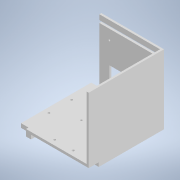
# Autodesk Inventor part: Quarter 3
Saved by Autodesk Inventor 2020.2 (Build 242310000, 310)
## iProperties
Created: 2020-01-17
Part Number: Quarter 3
Material: Generic
Document SubType Name: Modeling
Designer: ColinP
Density: 1 g/cm^3
Appearance: Default
Author: ColinP
Autodesk Inventor part; units mm, degrees
ref_plane "YZ Plane" through (0, 0, 0) normal (1, 0, 0) x (0, 1, 0)
ref_plane "XZ Plane" through (0, 0, 0) normal (0, 1, 0) x (-1, 0, 0)
ref_plane "XY Plane" through (0, 0, 0) normal (0, 0, 1) x (1, 0, 0)
sketch "Sketch1" plane through (0, 0, 0) normal (0, 1, 0) x (-1, 0, 0)
  line L0 (0, 0) -> (125, 0)
  line L1 (125, 0) -> (125, 150)
  line L2 (125, 150) -> (0, 150)
  line L3 (0, 150) -> (0, 0)
  dimension "d0" = 125
  dimension "d1" = 150
  constraints: 8 end point, 2 parallel, 1 horizontal, 1 perpendicular
  measures "d0" distance of L2.end L1.end
  measures "d1" distance of L1.end L0.end
extrude "Extrusion1" add sketch "Sketch1" along normal blind 10
sketch "Sketch2" plane through (0, 10, 0) normal (0, 1, 0) x (1, 0, 0)
  line L0 (-125, -150) -> (0, -150) projected
  line L1 (0, -150) -> (-4, -150)
  line L2 (-4, -150) -> (-4, -4)
  line L3 (-4, -4) -> (-125, -4)
  line L4 (-125, 0) -> (-125, -150) projected
  line L5 (0, -150) -> (0, 0) projected
  line L6 (0, 0) -> (-125, 0) projected
  line L7 (-125, 0) -> (-125, -150) projected
  line L8 (-125, -150) -> (0, -150) projected
  dimension "d4" = 4
  dimension "d5" = 146
  constraints: 6 end point, 2 perpendicular, 2 point on line
  measures "d4" distance of L0.end L1.end
  measures "d5" distance of L1.end L2.end
extrude "Extrusion2" add sketch "Sketch2" along normal blind 125 contours L2 L3 L4 L6 L5 L0
sketch "Sketch4" plane through (-125, 10, 4) normal (0, 0, 1) x (1, 0, 0)
  line L0 (0, -10) -> (0, 0) projected
  line L1 (0, 0) -> (0, 20)
  line L2 (0, -10) -> (0, 125) projected
  line L3 (0, 20) -> (20, 20)
  line L4 (20, 20) -> (86, 20)
  line L5 (86, 20) -> (86, 47)
  line L6 (86, 47) -> (20, 47)
  line L7 (20, 47) -> (20, 20)
  line L8 (20, 47) -> (20, 67)
  line L9 (20, 67) -> (20, 90)
  line L10 (20, 90) -> (20, 67)
  line L11 (20, 67) -> (81.6, 67)
  point P0 (125, -10)
  point P1 (0, -5)
  dimension "d11" = 20
  dimension "d12" = 20
  dimension "d13" = 66
  dimension "d14" = 27
  dimension "d15" = 20
  dimension "d55" = 23
  dimension "d56" = 61.6
  constraints: 20 end point, 3 horizontal, 3 perpendicular, 2 point on line, 1 collinear, 1 vertical
  measures "d11" distance of L0.end L1.end
  measures "d12" distance of L1.end L3.end
  measures "d13" distance of L3.end L4.end
  measures "d14" distance of L4.end L5.end
  measures "d15" distance of L6.end L8.end
  measures "d55" distance of L8.end L9.end
  measures "d56" distance of L8.end L11.end
extrude "Extrusion4" cut sketch "Sketch4" against normal blind 10
sketch "Sketch7" plane through (-125, 0, 150) normal (0, 0, 1) x (1, 0, 0)
  line L0 (125, 0) -> (0, 0) projected
  line L1 (125, 0) -> (125, 5)
  line L2 (125, 0) -> (125, 135) projected
  line L3 (125, 5) -> (10, 5)
  line L4 (10, 5) -> (10, 0)
  line L5 (10, 0) -> (125, 0)
  dimension "d32" = 5
  dimension "d33" = 115
  constraints: 8 end point, 2 perpendicular, 1 parallel, 1 point on line
  measures "d32" distance of L0.start L1.end
  measures "d33" distance of L1.end L3.end
extrude "Extrusion6" cut sketch "Sketch7" against normal blind 20
sketch "Sketch9" plane through (0, 0, 0) normal (0, -1, 0) x (1, 0, 0)
  line L0 (0, 130) -> (-115, 130) projected
  line L1 (0, 130) -> (-65, 130)
  line L2 (-65, 130) -> (-65, 80)
  line L3 (-65, 80) -> (-45, 80)
  line L4 (-45, 80) -> (-85, 80)
  point P0 (0, 0)
  dimension "d40" = 65
  dimension "d41" = 50
  dimension "d42" = 20
  dimension "d43" = 40
  constraints: 8 end point, 2 perpendicular, 2 point on line
  measures "d40" distance of L0.start L1.end
  measures "d41" distance of L1.end L2.end
  measures "d42" distance of L2.end L3.end
  measures "d43" distance of L3.end L4.end
hole "Hole2" at (-45, 0, 80) at (-85, 0, 80) direction (0, 1, 0) diameter 4 end through all counterbore diameter 6 counterbore depth 3
sketch "Sketch10" plane through (0, 135, 0) normal (0, 0, -1) x (-1, 0, 0)
  line L0 (0, 0) -> (125, 0) projected
  line L1 (125, 0) -> (125, -10)
  line L2 (125, -125) -> (125, 0) projected
  line L3 (125, -10) -> (4, -10)
  line L4 (4, -125) -> (4, 0) projected
  line L5 (4, -10) -> (4, -15)
  line L6 (4, -15) -> (125, -15)
  line L7 (125, -15) -> (125, -10)
  line L8 (125, -16.3986) -> (125, -10)
  line L9 (125, -10) -> (125, -15)
  point P0 (0, -135)
  dimension "d51" = 10
  dimension "d52" = 5
  constraints: 14 end point, 4 point on line, 3 perpendicular, 2 collinear, 1 vertical
  measures "d51" distance of L0.end L1.end
  measures "d52" distance of L3.end L5.end
extrude "Extrusion8" cut sketch "Sketch10" against normal blind 10 contours L3 L2 L6 L4
hole "Hole3" at (-105, 100, 4) at (-43.4, 77, 4) direction (0, 0, -1) diameter 3.5 end through all
sketch "Sketch12" plane through (-125, 0, 0) normal (-1, 0, 0) x (0, 0, 1)
  line L0 (150, 0) -> (140, 0)
  line L1 (140, 0) -> (140, 5)
  line L2 (150, 5) -> (130, 5) projected
  line L3 (140, 5) -> (0, 5)
  line L4 (0, 0) -> (0, 120) projected
  line L5 (0, 0) -> (0, 5)
  line L6 (4, 120) -> (0, 120) projected
  line L7 (0, 0) -> (0, 120) projected
  line L8 (0, 0) -> (150, 0) projected
  line L9 (150, 0) -> (150, 10) projected
  line L10 (4, 10) -> (150, 10) projected
  line L11 (4, 10) -> (4, 120) projected
  dimension "d77" = 10
  constraints: 8 end point, 1 collinear, 1 horizontal, 1 midpoint, 1 perpendicular, 1 point on line
  measures "d77" distance of L0.start L0.end
extrude "Extrusion9" add sketch "Sketch12" along normal blind 20 contours L8 L4 L3 L2 L1
sketch "Sketch11" plane through (0, 10, 0) normal (0, 1, 0) x (1, 0, 0)
  line L0 (-115, -150) -> (-115, -130) projected
  line L1 (-115, -150) -> (-78, -150)
  line L2 (-125, -150) -> (-4, -150) projected
  line L3 (-78, -150) -> (-78, -140)
  line L4 (-78, -140) -> (-41, -140)
  line L5 (-125, -140) -> (-125, -150) projected
  line L6 (-125, -140) -> (-125, -94.6667)
  line L7 (-125, -4) -> (-125, -150) projected
  line L8 (-125, -94.6667) -> (-135, -94.6667)
  line L9 (-135, -94.6667) -> (-135, -49.3333)
  point P0 (0, 0)
  dimension "d67" = 37
  dimension "d68" = 10
  dimension "d69" = 37
  dimension "d80" = 45.3333
  dimension "d81" = 45.3333
  constraints: 12 end point, 4 perpendicular, 2 point on line
  measures "d67" distance of L0.start L1.end
  measures "d68" distance of L1.end L3.end
  measures "d69" distance of L3.end L4.end
  measures "d80" distance of L5.start L6.end
  measures "d81" distance of L8.end L9.end
hole "Hole4" at (-78, 10, 140) at (-41, 10, 140) direction (0, -1, 0) diameter 4.318 end through all
hole "Hole5" at (-135, 10, 94.6667) at (-135, 10, 49.3333) direction (0, -1, 0) diameter 3.5 end through all
sketch "Sketch13" plane through (0, 0, 0) normal (0, -1, 0) x (1, 0, 0)
  circle A0 centre (-135, 94.6667) radius 1.75 projected
  circle A1 centre (-135, 49.3333) radius 1.75 projected
  circle A2 centre (-45, 80) radius 3 projected
  circle A3 centre (-85, 80) radius 3 projected
  line L0 (0, 130) -> (-115, 130) projected
  line L1 (-115, 130) -> (-115, 150) projected
  line L2 (-125, 150) -> (-115, 150) projected
  line L3 (-125, 140) -> (-125, 150) projected
  line L4 (-125, 140) -> (-145, 140) projected
  line L5 (-145, 0) -> (-145, 140) projected
  line L6 (0, 0) -> (-145, 0) projected
  line L7 (0, 130) -> (0, 0) projected
extrude "Extrusion10" add sketch "Sketch13" along normal blind 3
sketch "Sketch14" plane through (-45, 3, 80) normal (0, -1, 0) x (1, 0, 0)
  circle A0 centre (0, 0) radius 3 projected
  circle A1 centre (0, 0) radius 2 projected
  circle A2 centre (-40, 0) radius 3 projected
  circle A3 centre (-40, 0) radius 2 projected
  point P0 (45, -80)
extrude "Extrusion11" add sketch "Sketch14" along normal blind 3
sketch "Sketch15" plane through (0, -3, 0) normal (0, -1, 0) x (1, 0, 0)
  circle A0 centre (-135, 49.3333) radius 1.75 projected
  circle A1 centre (-135, 94.6667) radius 1.75 projected
  point P0 (0, 0)
hole "Hole6" at (-135, -3, 94.6667) at (-135, -3, 49.3333) direction (0, 1, 0) diameter 4.318 end through all counterbore diameter 7.62 counterbore depth 5.08
body "Solid1"
